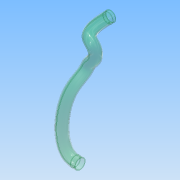
# Autodesk Inventor part: Top_Lower Pipe 7
Saved by Autodesk Inventor 2018.1 (Build 221171000, 171)
## iProperties
Created: 2019-03-21
Part Number: Top_Lower Pipe 7
Material: PMMA Plastic
Document SubType Name: Modeling
Designer: James
Density: 1.188 g/cm^3
Appearance: Clear - Green 1
Author: James
Autodesk Inventor part; units mm, degrees
ref_plane "YZ Plane" through (0, 0, 0) normal (1, 0, 0) x (0, 1, 0)
ref_plane "XZ Plane" through (0, 0, 0) normal (0, 1, 0) x (-1, 0, 0)
ref_plane "XY Plane" through (0, 0, 0) normal (0, 0, 1) x (1, 0, 0)
sketch "Sketch2" plane through (0, 0, 0) normal (0, 1, 0) x (-1, 0, 0)
  circle A0 centre (0, 0) radius 23
  circle A1 centre (0, 0) radius 20
  dimension "d1" = 46
  dimension "d2" = 40
  constraints: 2 centre point, 2 coincident
  measures "d1" diameter of A0
  measures "d2" diameter of A1
sketch3d "3D Sketch1"
  spline S0 degree 4 poles (0, 0, 0) (0, -117, 0) (70, -117, 0) (70, -117, -80) (30, -117, -80) (30, -117, -145) (30, -242, -145) (30, -242, -368) (101, -242, -368) knots 1 1 1 1 1 2 3 4 5 6 6 6 6 6
  dimension "d31" = 117
  dimension "d32" = 70
  dimension "d33" = 80
  dimension "d34" = 40
  dimension "d35" = 65
  dimension "d36" = 125
  dimension "d37" = 223
  dimension "d38" = 71
sweep "Sweep1" add profiles "Sketch2" path "3D Sketch1"
sketch "Sketch3" plane through (0, 0, 0) normal (0, 1, 0) x (1, 0, 0)
  spline S0 degree 6 poles (-20, 0) (-20, 33.2309) (21.091, 38.0022) (54.9823, 0) (21.091, -38.0022) (-20, -33.2309) (-20, 0) knots 0 0 0 0 0 0 0 1 1 1 1 1 1 1 weights 1.669078 1.03673 1.038347 0.853534 1.038347 1.03673 1.669078 projected
  circle A0 centre (0, 0) radius 23 projected
  point P0 (-23, 0)
  constraints: 1 horizontal alignment, 1 other
extrude "Extrusion1" add sketch "Sketch3" along normal blind 12
sketch "Sketch4" plane through (0, 0, 0) normal (0, 0, 1) x (1, 0, 0)
  line L0 (23, 12) -> (-23, 12) projected
  point P0 (0, 0)
  point P1 (0, 5)
  point P2 (0, 12)
  dimension "d11" = 7
  constraints: 1 midpoint, 1 vertical alignment
  measures "d11" distance from line of L0 point (0, 5)
hole "Hole1" at (0, 5, 0) direction (0, 0, -1) diameter 4.5 end through all
sketch "Sketch5" plane through (101, -242, -368) normal (1, 0, 0) x (0, 0, -1)
  spline S0 degree 6 poles (1.6127, -19.9349) (34.7354, -17.2553) (36.1778, 24.0866) (-4.4335, 54.8033) (-39.5792, 17.958) (-31.5099, -22.6145) (1.6127, -19.9349) knots 0 0 0 0 0 0 0 1 1 1 1 1 1 1 weights 1.669078 1.03673 1.038347 0.853534 1.038347 1.03673 1.669078 projected
  circle A0 centre (0, 0) radius 23 projected
  point P0 (-368, 242)
  point P1 (1.9041, -22.921)
  constraints: 2 other
extrude "Extrusion2" add sketch "Sketch5" along normal blind 20
body "Solid1"
